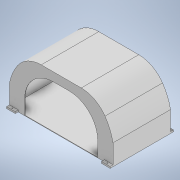
# Autodesk Inventor part: COVER,711
Saved by Autodesk Inventor 2020 (Build 240168000, 168)
## iProperties
Created: 2021-05-02
Part Number: COVER,711
Material: Generic
Document SubType Name: Modeling
Designer: Hengameh
Density: 1 g/cm^3
Appearance: Default
Author: Hengameh
Autodesk Inventor part; units mm, degrees
ref_plane "YZ Plane" through (0, 0, 0) normal (1, 0, 0) x (0, 1, 0)
ref_plane "XZ Plane" through (0, 0, 0) normal (0, 1, 0) x (-1, 0, 0)
ref_plane "XY Plane" through (0, 0, 0) normal (0, 0, 1) x (1, 0, 0)
sketch "Sketch1" plane through (0, 0, 0) normal (0, 0, 1) x (1, 0, 0)
  line L0 (-900, 0) -> (900, 0)
  line L1 (900, 0) -> (900, 900)
  line L2 (900, 900) -> (-900, 900)
  line L3 (-900, 900) -> (-900, 0)
  line L4 (0, 900) -> (0, 0) construction
  dimension "d0" = 900
  dimension "d1" = 1800
  constraints: 10 end point, 2 midpoint, 2 parallel, 1 coincident, 1 horizontal, 1 perpendicular
  measures "d0" distance of L2.end L0.start
  measures "d1" distance of L1.end L2.end
extrude "Extrusion1" add sketch "Sketch1" along normal mid plane 1000
sketch "Sketch2" plane through (0, 0, 500) normal (0, 0, 1) x (1, 0, 0)
  line L0 (-900, 900) -> (-900, 0) projected
  arc A0 (-550, 900) -> (-900, 350) centre (-17.254, 174.6162) ccw
  line L1 (900, 900) -> (-900, 900) projected
  line L2 (-900, 350) -> (-900, 900)
  line L3 (-900, 900) -> (-550, 900)
  point P0 (0, 0)
  dimension "d5" = 900
  dimension "d6" = 550
  dimension "d7" = 350
  constraints: 4 end point, 2 point on circle, 2 point on line, 1 centre point, 1 collinear
  measures "d5" radius of A0
  measures "d6" distance from line of L2.start L1
  measures "d7" distance of L3.end L0.start
extrude "Extrusion2" cut sketch "Sketch2" against normal blind 1000
mirror "Mirror1" about plane through (0, 0, 0) normal (1, 0, 0) of "Extrusion2"
fillet "Fillet1" radius 500 2 edges at (-550, 900, 0) (550, 900, 0)
sketch "Sketch3" plane through (0, 0, 500) normal (0, 0, 1) x (1, 0, 0)
  arc A0 (-347.7115, 900) -> (-760.7833, 681.7298) centre (-347.7115, 400) ccw projected
  line L0 (347.7115, 900) -> (-347.7115, 900) projected
  arc A1 (760.7833, 681.7298) -> (347.7115, 900) centre (347.7115, 400) ccw projected
  arc A2 (-347.7115, 750) -> (-634.9396, 600) centre (-347.7115, 400) ccw
  line L1 (-347.7115, 750) -> (347.7115, 750)
  arc A3 (634.9396, 600) -> (347.7115, 750) centre (347.7115, 400) ccw
  line L2 (-634.9396, 600) -> (-634.9396, 0)
  line L3 (900, 0) -> (-900, 0) projected
  line L4 (634.9396, 600) -> (634.9396, 0)
  line L5 (634.9396, 0) -> (-634.9396, 0)
  point P0 (0, 0)
  point P1 (634.9396, 0)
  dimension "d11" = 150
  dimension "d12" = 600
  constraints: 8 end point, 4 point on circle, 2 centre point, 2 vertical, 1 parallel, 1 perpendicular, 1 point on line, 2 other
  measures "d11" distance between parallel lines of L0 L1
  measures "d12" distance of L2.start L2.end
shell "Shell2" thickness 5 removed faces 1 at (300, 0, 166.6667)
extrude "Extrusion3" cut sketch "Sketch3" against normal blind 10
fillet "Fillet2" radius 500 2 edges at (-634.9396, 600, 497.5) (634.9396, 600, 497.5)
sketch "Sketch4" plane through (-900, 0, -500) normal (0, -1, 0) x (1, 0, 0)
  line L0 (1534.9396, 1000) -> (1800, 1000) projected
  line L1 (0, 0) -> (1800, 0)
  line L2 (1800, 0) -> (1800, 1000)
  line L3 (1800, 1000) -> (0, 1000)
  line L4 (0, 1000) -> (0, 0)
  point P0 (900, 500)
  constraints: 8 end point, 2 parallel, 1 horizontal, 1 perpendicular
extrude "Extrusion4" add sketch "Sketch4" along normal blind 10
sketch "Sketch5" plane through (0, 0, 500) normal (0, 0, 1) x (1, 0, 0)
  line L0 (-900, -10) -> (900, -10) projected
  line L1 (-900, -10) -> (-750, -10)
  line L2 (-750, -10) -> (-750, 20)
  line L3 (-750, 20) -> (-900, 20)
  line L4 (-900, 20) -> (-900, -10)
  line L5 (900, -10) -> (750, -10)
  line L6 (750, -10) -> (750, 20)
  line L7 (750, 20) -> (900, 20)
  line L8 (900, 20) -> (900, -10)
  point P0 (0, 0)
  dimension "d19" = 30
  dimension "d20" = 150
  dimension "d21" = 30
  dimension "d22" = 150
  constraints: 16 end point, 4 parallel, 2 horizontal, 2 perpendicular
  measures "d19" distance of L3.end L0.start
  measures "d20" distance between parallel lines of L2 L4
  measures "d21" distance of L7.end L0.end
  measures "d22" distance of L6.end L7.end
extrude "Extrusion5" add sketch "Sketch5" along normal blind 50
sketch "Sketch6" plane through (-900, 20, 500) normal (0, 1, 0) x (1, 0, 0)
  circle A0 centre (75, -25) radius 8
  circle A1 centre (1725, -25) radius 8
  line L0 (75, -25) -> (1725, -25) construction
  line L1 (1800, -50) -> (1650, -50) construction
  line L2 (1650, 0) -> (1650, -50) construction
  line L3 (0, 0) -> (0, -50) construction
  point P0 (900, 500)
  dimension "d25" = 16
  dimension "d26" = 25
  dimension "d27" = 75
  dimension "d28" = 75
  constraints: 2 centre point, 2 end point, 1 equal radius, 1 horizontal
  measures "d25" diameter of A1
  measures "d26" distance between parallel lines of L1 L0
  measures "d27" distance from line of L2 L0.end
  measures "d28" distance from line of L3 L0.start
extrude "Extrusion6" cut sketch "Sketch6" against normal blind 50
mirror "Mirror2" about plane through (0, 0, 0) normal (0, 0, 1) of "Extrusion6", "Extrusion5"
ref_plane "Work Plane1" through (0, 0, 0) normal (1, 0, 0) x (0, 1, 0)
equation "\"d0\" = 0.5 * d1"
body "Solid1"
